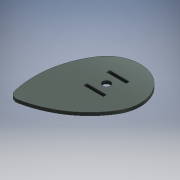
# Autodesk Inventor part: leva00
Saved by Autodesk Inventor 2016 (Build 200138000, 138)
## iProperties
Created: 2016-09-20
Part Number: leva00
Material: Madera (abedul)
Document SubType Name: Modeling
Designer: i95sa
Density: 0.55 g/cm^3
Appearance: Gris plomo - Pulido
Author: i95sa
Autodesk Inventor part; units mm, degrees
ref_plane "YZ Plane" through (0, 0, 0) normal (1, 0, 0) x (0, 1, 0)
ref_plane "XZ Plane" through (0, 0, 0) normal (0, 1, 0) x (-1, 0, 0)
ref_plane "XY Plane" through (0, 0, 0) normal (0, 0, 1) x (1, 0, 0)
sketch "Boceto1" plane through (0, 0, 0) normal (0, 0, 1) x (1, 0, 0)
  arc A0 (23.1263, 36.4412) -> (-23.1263, -36.4412) centre (0, 0) ccw
  arc A1 (-35.5895, -56.0801) -> (-46.2632, -72.8991) centre (-40.9264, -64.4896) ccw
  line L0 (-47.8084, -75.3339) -> (-56.2179, -69.9971)
  line L1 (-36.1647, 23.5563) -> (-50.1805, 32.4511)
  line L2 (-50.1805, 32.4511) -> (-56.2179, -69.9971)
  line L3 (-56.2179, -69.9971) -> (-53.8741, -30.2261)
  arc A2 (-36.1647, 23.5563) -> (-53.8741, -30.2261) centre (56.3793, -36.7234) ccw
  arc A3 (-53.8741, -30.2261) -> (-50.6083, -66.8267) centre (70.6269, -37.563) ccw
  line L4 (1.7789, 2.8032) -> (23.1263, 36.4412)
  line L5 (-1.7789, -2.8032) -> (-47.8084, -75.3339)
  arc A4 (-23.1263, -36.4412) -> (23.1263, 36.4412) centre (0, 0) ccw
  arc A5 (-46.2632, -72.8991) -> (-35.5895, -56.0801) centre (-40.9264, -64.4896) ccw
  line L6 (-47.8084, -75.3339) -> (-39.3988, -80.6707)
  line L7 (36.7126, -22.693) -> (50.7284, -31.5877)
  line L8 (50.7284, -31.5877) -> (-39.3988, -80.6707)
  line L9 (-39.3988, -80.6707) -> (-4.4109, -61.6164)
  arc A6 (-4.4109, -61.6164) -> (36.7126, -22.693) centre (-57.2334, 35.3774) ccw
  arc A7 (-38.9186, -74.2452) -> (-4.4109, -61.6164) centre (-64.0595, 47.9116) ccw
  dimension "d0" = 86.32
  dimension "d6" = 19.92
  dimension "d7" = 9.96
  dimension "d8" = 16.6
  dimension "d9" = 39.84
  constraints: 20 end point, 20 point on circle, 8 centre point, 6 symmetric about line, 5 point on line, 4 tangent, 1 collinear, 4 other
  measures "d0" diameter of A0
  measures "d6" diameter of A1
  measures "d7" distance of L0.start L0.end
  measures "d8" distance of L1.start L1.end
  measures "d9" distance of L0.end L3.end
extrude "Extrusión2" add sketch "Boceto1" along normal blind 4 contours A4 A0 | A0 L5 A1 A3 A2 | A6 A7 A5 L5 A4 | L5 A1 | A5 L5
sketch "Boceto2" plane through (0, 0, 4) normal (0, 0, 1) x (1, 0, 0)
  line L0 (0, 0) -> (0, 12.5)
  line L1 (0, 12.5) -> (-12.5, 12.5)
  line L2 (-12.5, 12.5) -> (-12.5, 16.7)
  line L3 (-12.5, 16.7) -> (12.5, 16.7)
  line L4 (12.5, 16.7) -> (12.5, 12.5)
  line L5 (12.5, 12.5) -> (0, 12.5)
  line L6 (0, 0) -> (12.5, 0)
  line L7 (0, 0) -> (0, -12.5)
  line L8 (0, -12.5) -> (-12.5, -12.5)
  line L9 (-12.5, -12.5) -> (-12.5, -16.7)
  line L10 (-12.5, -16.7) -> (12.5, -16.7)
  line L11 (12.5, -16.7) -> (12.5, -12.5)
  line L12 (12.5, -12.5) -> (0, -12.5)
  circle A0 centre (0, 0) radius 5
  dimension "d24" = 12.5
  dimension "d25" = 12.5
  dimension "d26" = 4.2
  dimension "d27" = 25
  dimension "d28" = 10
  constraints: 26 end point, 5 perpendicular, 5 symmetric about line, 3 point on line, 1 centre point, 1 coincident, 1 parallel, 1 vertical
  measures "d24" distance of L0.start L0.end
  measures "d25" distance of L0.end L1.end
  measures "d26" distance of L1.end L2.end
  measures "d27" distance of L2.end L3.end
  measures "d28" diameter of A0
extrude "Extrusión3" cut sketch "Boceto2" against normal blind 4
